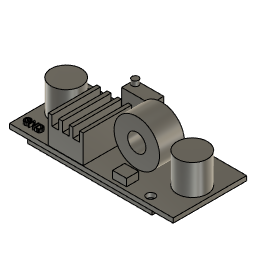
18650 Dual Battery Handle 5A Reg v20 (Autodesk Fusion 360 archive; units mm, degrees)
design "Buck Regulator 5A"
Autodesk Fusion 360 part; units mm, degrees
sketch "caps and trimmer" plane through (0, 0, 0) normal (0, 0, 1) x (1, 0, 0)
  line L0 (0, 0) -> (54, 0)
  line L1 (54, 0) -> (54, 24.2)
  line L2 (54, 24.2) -> (0, 24.2)
  line L3 (0, 24.2) -> (0, 0)
  dimension "d1" = 54
  dimension "d2" = 24.2
  constraint horizontal L0
  constraint vertical L1
  constraint horizontal L2
  constraint vertical L3
  constraint coincident L0.start L3.end
  measures "d1" distance of L0.start L0.end
  measures "d2" distance of L0.start L2.end
extrude "Extrude1" add sketch "caps and trimmer" along normal blind 1.5 makes body 1
hole "Hole1" at (9, 21.6, 1.5) direction (0, 0, -1) diameter 2.8 end up to surface (1.5 mm away) bodies 1
hole "Hole2" at (44, 2.6, 1.5) direction (0, 0, -1) diameter 2.8 end up to surface (1.5 mm away) bodies 1
sketch "reg chip" plane through (0, 0, 1.5) normal (0, 0, 1) x (-1, 0, 0)
  circle A0 centre (-44, -2.6) radius 1.4
  circle A1 centre (-9, -21.6) radius 1.4
  line L0 (0, -24.2) -> (0, 0)
  line L1 (0, 0) -> (-54, 0)
  line L2 (-54, 0) -> (-54, -24.2)
  line L3 (-54, -24.2) -> (0, -24.2)
  circle A2 centre (-6.2, -12.5) radius 5
  circle A3 centre (-47.8, -12.5) radius 5
  line L4 (-18.2, -23.2) -> (-27.7, -23.2)
  line L5 (-27.7, -23.2) -> (-27.7, -18.8)
  line L6 (-27.7, -18.8) -> (-18.2, -18.8)
  line L7 (-18.2, -18.8) -> (-18.2, -23.2)
  line L8 (-12.7, -16.1) -> (-24.2, -16.1)
  line L9 (-24.2, -16.1) -> (-24.2, -0.1)
  line L10 (-24.2, -0.1) -> (-12.7, -0.1)
  line L11 (-12.7, -0.1) -> (-12.7, -16.1)
  line L12 (-32.8, -5.2) -> (-37.4, -5.2)
  line L13 (-37.4, -5.2) -> (-37.4, -1.2)
  line L14 (-37.4, -1.2) -> (-32.8, -1.2)
  line L15 (-32.8, -1.2) -> (-32.8, -5.2)
  dimension "d15" = 10
  dimension "d16" = 6.2
  dimension "d17" = 12.5
  dimension "d18" = 10
  dimension "d19" = 6.2
  dimension "d20" = 12.5
  dimension "d23" = 9.5
  dimension "d24" = 4.4
  dimension "d25" = 1
  dimension "d26" = 18.2
  dimension "d30" = 11.5
  dimension "d31" = 16
  dimension "d32" = 0.1
  dimension "d33" = 12.7
  dimension "d44" = 4.6
  dimension "d45" = 4
  dimension "d46" = 16.6
  dimension "d47" = 1.2
  constraint horizontal L4
  constraint vertical L5
  constraint horizontal L6
  constraint vertical L7
  constraint horizontal L8
  constraint vertical L9
  constraint horizontal L10
  constraint vertical L11
  constraint horizontal L12
  constraint vertical L13
  constraint horizontal L14
  constraint vertical L15
  measures "d15" diameter of A2
  measures "d16" distance of L0 A2.centre
  measures "d17" distance of L1 A2.centre
  measures "d18" diameter of A3
  measures "d19" distance of L2 A3.centre
  measures "d20" distance of L1 A3.centre
  measures "d23" distance of L4.start L4.end
  measures "d24" distance of L4.start L6.end
  measures "d25" distance of L3 L4
  measures "d26" distance of L0 L7
  measures "d30" distance of L8.start L8.end
  measures "d31" distance of L8.start L10.end
  measures "d32" distance of L1 L10
  measures "d33" distance of L0 L11
  measures "d44" distance of L12.start L12.end
  measures "d45" distance of L12.start L14.end
  measures "d46" distance of L2 L13
  measures "d47" distance of L1 L14
extrude "Extrude6" add sketch "reg chip" along normal blind 2.4 contours L12 L13 L14 L15 bodies 1
extrude "Extrude2" add sketch "reg chip" along normal blind 10 contours A2 | A3 | L4 L5 L6 L7 bodies 1
sketch "trimmer screw" plane through (0, 0, 11.5) normal (0, 0, 1) x (-1, 0, 0)
  line L0 (-18.2, -18.8) -> (-27.7, -18.8)
  line L1 (-27.7, -18.8) -> (-27.7, -23.2)
  line L2 (-27.7, -23.2) -> (-18.2, -23.2)
  line L3 (-18.2, -23.2) -> (-18.2, -18.8)
  circle A0 centre (-19.456, -22.017) radius 1.1
  dimension "d27" = 2.2
  measures "d27" diameter of A0
extrude "Extrude3" add sketch "trimmer screw" along normal blind 1.6 contours A0 bodies 1
extrude "Extrude4" add sketch "reg chip" along normal blind 9.3 contours L8 L9 L10 L11 bodies 1
ref_plane "WorkPlane1" through (27, 12.1, 0.75) normal (0, 1, 0) x (-1, 0, 0)
sketch "toroid" plane through (27, 12.1, 0.75) normal (0, 1, 0) x (1, 0, 0)
  circle A0 centre (7, -8.25) radius 7.5
  line L0 (-27, -0.75) -> (27, -0.75)
  dimension "d36" = 15
  dimension "d37" = 7.5
  dimension "d38" = 20
  measures "d36" diameter of A0
  measures "d37" distance of A0.centre L0
  measures "d38" horizontal distance of A0.centre L0.end
extrude "Extrude5" add sketch "toroid" along normal mid plane 8.2 separate body makes body 2
hole "Hole3" at (34, 8, 9) direction (0, 1, 0) diameter 6 end up to surface (8.2 mm away) bodies 2
sketch "heat sink fins" plane through (0, 0.1, 0) normal (0, -1, 0) x (1, 0, 0)
  line L0 (12.7, 1.5) -> (24.2, 1.5)
  line L1 (24.2, 1.5) -> (24.2, 10.8)
  line L2 (24.2, 10.8) -> (12.7, 10.8)
  line L3 (12.7, 10.8) -> (12.7, 1.5)
  line L4 (13.9, 10.8) -> (16.1, 10.8)
  line L5 (16.1, 10.8) -> (16.1, 7.6)
  line L6 (16.1, 7.6) -> (13.9, 7.6)
  line L7 (13.9, 7.6) -> (13.9, 10.8)
  line L8 (23, 7.6) -> (20.8, 7.6)
  line L9 (23, 10.8) -> (23, 7.6)
  line L10 (20.8, 7.6) -> (20.8, 10.8)
  line L11 (17.4, 10.8) -> (19.6, 10.8)
  line L12 (19.6, 10.8) -> (19.6, 7.6)
  line L13 (19.6, 7.6) -> (17.4, 7.6)
  line L14 (17.4, 7.6) -> (17.4, 10.8)
  dimension "d50" = 2.2
  dimension "d51" = 3.2
  dimension "d52" = 1.2
  dimension "d53" = 2.2
  dimension "d54" = 1.2
  dimension "d55" = 3.2
  dimension "d56" = 2.2
  dimension "d57" = 3.2
  constraint horizontal L4
  constraint vertical L5
  constraint horizontal L6
  constraint vertical L7
  constraint coincident L2 L4.start
  constraint vertical L9
  constraint horizontal L8
  constraint vertical L10
  constraint horizontal L11
  constraint vertical L12
  constraint horizontal L13
  constraint vertical L14
  measures "d50" distance of L5 L7
  measures "d51" distance of L4 L6
  measures "d52" distance of L3 L7
  measures "d53" distance of L9 L10
  measures "d54" distance of L1 L9
  measures "d55" distance of L2 L8
  measures "d56" distance of L12 L14
  measures "d57" distance of L11 L13
extrude "Extrude7" cut sketch "heat sink fins" against normal up to surface (16 mm away) contours L2 L4 L5 L6 L7 | L2 L8 L9 L10 | L2 L11 L12 L13 L14 bodies 1
sketch "text" plane through (0, 0, 1.5) normal (0, 0, 1) x (-1, 0, 0)
  line L0 (-12.7, -0.1) -> (-12.7, -16.1)
  line L1 (-12.7, -16.1) -> (-24.2, -16.1)
  line L2 (-24.2, -16.1) -> (-24.2, -0.1)
  line L3 (-24.2, -0.1) -> (-12.7, -0.1)
  line L4 (-18.2, -18.8) -> (-18.2, -23.2)
  line L5 (-18.2, -23.2) -> (-27.7, -23.2)
  line L6 (-27.7, -23.2) -> (-27.7, -18.8)
  line L7 (-27.7, -18.8) -> (-18.2, -18.8)
  circle A0 centre (-6.2, -12.5) radius 5
  circle A1 centre (-47.8, -12.5) radius 5
  line L8 (-32.8, -1.2) -> (-32.8, -5.2)
  line L9 (-32.8, -5.2) -> (-37.4, -5.2)
  line L10 (-37.4, -5.2) -> (-37.4, -1.2)
  line L11 (-37.4, -1.2) -> (-32.8, -1.2)
  circle A2 centre (-44, -2.6) radius 1.4
  circle A3 centre (-9, -21.6) radius 1.4
  line L12 (0, -24.2) -> (0, 0)
  line L13 (0, 0) -> (-54, 0)
  line L14 (-54, 0) -> (-54, -24.2)
  line L15 (-54, -24.2) -> (0, -24.2)
  line L16 (-2, -20) -> (-6, -20) construction
  line L17 (-6, -20) -> (-6, -22) construction
  line L18 (-6, -22) -> (-2, -22) construction
  line L19 (-2, -22) -> (-2, -20) construction
  line L20 (-2, -2) -> (-6, -2) construction
  line L21 (-6, -2) -> (-6, -4) construction
  line L22 (-6, -4) -> (-2, -4) construction
  line L23 (-2, -4) -> (-2, -2) construction
  dimension "d60" = 2
  dimension "d61" = 2
  text T0 "IN+" font "Arial" height 2 align left top in box 4 x 2 at (-2, -20) x (-1, 0) y (0, -1) spacing 1 kerned
  text T1 "GND" font "Arial" height 2 align left top in box 4 x 2 at (-2, -2) x (-1, 0) y (0, -1) spacing 1 kerned
extrude "Extrude8" add sketch "text" along normal blind 1 text T1 T0 bodies 1
sketch "Sketch1" plane through (0, 0, 0) normal (0, 0, 1) x (1, 0, 0) in component "shim"
  line L0 (6, 24) -> (47, 24)
  line L1 (47, 24) -> (47, 0)
  line L2 (47, 0) -> (6, 0)
  line L3 (6, 0) -> (6, 24)
  circle A0 centre (9.0325, 21.589) radius 1.6
  circle A1 centre (44.0105, 2.5723) radius 1.6
  line L4 (17, 24) -> (17, 3)
  line L5 (17, 3) -> (40, 3)
  line L6 (40, 3) -> (40, 24)
  dimension "d64" = 24
  dimension "d65" = 41
  dimension "d66" = 3.2
  dimension "d67" = 3.2
  dimension "d68" = 21
  dimension "d69" = 23
  dimension "d70" = 21
  constraint horizontal L0
  constraint vertical L1
  constraint horizontal L2
  constraint vertical L3
  constraint coincident L0 L4.start
  constraint perpendicular L0 L4
  constraint perpendicular L4 L5
  constraint perpendicular L0 L6
  measures "d64" distance of L0 L2
  measures "d65" distance of L1 L3
  measures "d66" diameter of A0
  measures "d67" diameter of A1
  measures "d68" distance of L4.start L4.end
  measures "d69" distance of L4.end L5.end
  measures "d70" distance of L5.end L6.end
extrude "Extrude1'" add sketch "Sketch1" along normal blind 1.2 separate body contours L0 L1 L2 L3 L4 L5 L6 makes body 3 in component "shim"
component "shim" placed x (1, 0, 0) y (0, 1, 0) z (0, 0, 1) at (0, 0, -1.2)
